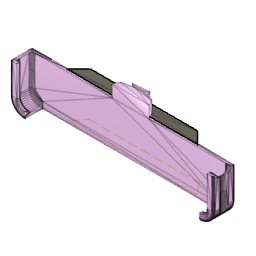
MotoZ3 case (Autodesk Fusion 360 design; units mm, degrees)
Autodesk Fusion 360 part; units mm, degrees
mesh "Mesh1" [no effect]
sketch "Sketch1" plane through (0, 0, 0) normal (0, 0, 1) x (1, 0, 0)
  line L0 (31.5174, 2.3764) -> (38.4719, 11.4025) construction
  line L1 (38.4719, 11.4025) -> (130, 11.4025) construction
  line L2 (130, 11.4025) -> (138.3507, 1.4886) construction
  line L3 (138.3507, 1.4886) -> (30.8333, 1.4886) construction
  line L4 (30.8333, 1.4886) -> (31.5174, 2.3764) construction
  constraint horizontal L1
  constraint parallel L1 L3
  constraint parallel L0 L4
sketch "Sketch2" plane through (0, 0, 0) normal (0, 0, 1) x (1, 0, 0)
  line L0 (30.0881, 1.5936) -> (138.6299, 1.5936)
  line L1 (128.8668, 11.3566) -> (39.8511, 11.3566)
  line L2 (30.0881, 1.5936) -> (39.8511, 11.3566)
  line L3 (138.6299, 1.5936) -> (128.8668, 11.3566)
  constraint horizontal L0
  constraint horizontal L1
  constraint perpendicular L2 L3
extrude "Extrude1" add sketch "Sketch2" along normal blind 37
